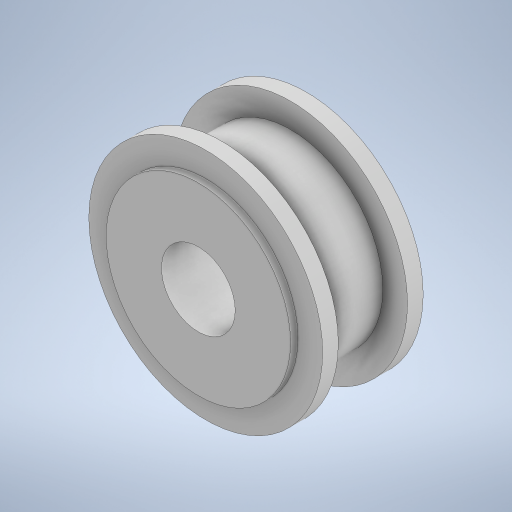
# Autodesk Inventor part: timing _pulley_7.5_8
Saved by Autodesk Inventor 2023 (Build 270158000, 158)
## iProperties
Created: 2022-12-09
Part Number: timing _pulley_7.5_8
Material: 一般
Document SubType Name: Modeling
Designer: zegi
Density: 1 g/cm^3
Appearance: 既定
Author: zegi
Autodesk Inventor part; units mm, degrees
ref_plane "YZ Plane" through (0, 0, 0) normal (1, 0, 0) x (0, 1, 0)
ref_plane "XZ Plane" through (0, 0, 0) normal (0, 1, 0) x (-1, 0, 0)
ref_plane "XY Plane" through (0, 0, 0) normal (0, 0, 1) x (1, 0, 0)
sketch "スケッチ1" plane through (0, 0, 0) normal (0, 0, 1) x (1, 0, 0)
  circle A0 centre (0, 0) radius 12.675
  circle A1 centre (0, 0) radius 4
  circle A2 centre (0, 0) radius 10
  circle A3 centre (0, 0) radius 16
  dimension "d0" = 25.35
  dimension "d1" = 8
  dimension "d2" = 20
  dimension "d3" = 32
  constraints: 4 centre point, 4 coincident
  measures "d0" diameter of A0
  measures "d1" diameter of A1
  measures "d2" diameter of A2
  measures "d3" diameter of A3
extrude "押し出し1" add sketch "スケッチ1" along normal blind 3.75 contours A2
extrude "押し出し2" add sketch "スケッチ1" against normal blind 1.7 contours A0
extrude "押し出し3" add sketch "スケッチ1" against normal blind 2.5 contours A2
mirror "ミラー1" about plane through (0, 0, 3.75) normal (0, 0, 1) of "押し出し1", "押し出し2", "押し出し3"
